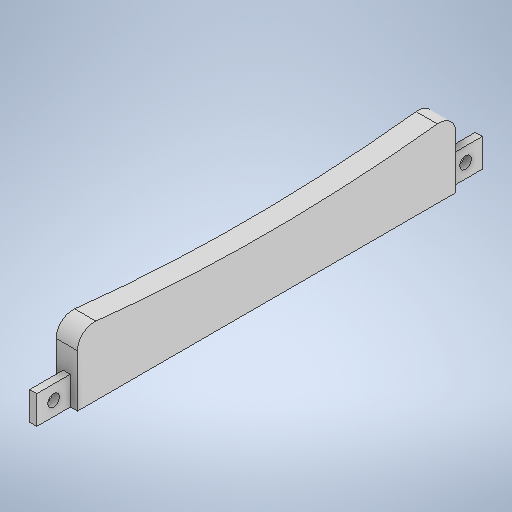
# Autodesk Inventor part: FretBar
Saved by Autodesk Inventor 2025.1 (Build 291241000, 241)
## iProperties
Created: 2025-12-10
Part Number: FretBar
Material: Generic
Document SubType Name: Modeling
Designer: Juxin
Density: 1 g/cm^3
Appearance: Default
Author: Juxin
Title: Fret Bar
Autodesk Inventor part; units mm, degrees
ref_plane "YZ Plane" through (0, 0, 0) normal (1, 0, 0) x (0, 1, 0)
ref_plane "XZ Plane" through (0, 0, 0) normal (0, 1, 0) x (-1, 0, 0)
ref_plane "XY Plane" through (0, 0, 0) normal (0, 0, 1) x (1, 0, 0)
sketch "Sketch1" plane through (0, 0, 0) normal (0, 1, 0) x (-1, 0, 0)
  line L0 (0, 0) -> (1.905, 0)
  line L1 (1.905, -119.6501) -> (0, -119.6501)
  line L2 (0, 0) -> (0, -9.025)
  line L3 (0, 0) -> (9.025, 0) construction
  line L4 (0, -9.025) -> (1.905, -9.025)
  line L5 (0, -119.6501) -> (0, -110.625)
  line L6 (0, -110.625) -> (1.905, -110.625)
  line L7 (1.905, -9.025) -> (3.81, -9.025)
  line L8 (3.81, -9.025) -> (3.81, -110.625)
  line L9 (3.81, -110.625) -> (1.905, -110.625)
  line L10 (0, -9.025) -> (-1.905, -9.025)
  line L11 (-1.905, -9.025) -> (-1.905, -110.625)
  line L12 (-1.905, -110.625) -> (0, -110.625)
  line L13 (1.905, 0) -> (1.905, -9.025)
  line L14 (1.905, -110.625) -> (1.905, -119.6501)
  line L15 (0, -119.6501) -> (0, -110.625)
  line L16 (0, -9.025) -> (0, 0)
  dimension "d19" = 101.6
  dimension "d20" = 1.905
  dimension "d21" = 1.905
  dimension "d22" = 1.905
  dimension "d23" = 1.905
  dimension "d24" = 1.905
  dimension "d25" = 1.905
  constraints: 34 end point, 11 equal length, 9 perpendicular, 4 horizontal, 1 point on line
  measures "d19" distance of L10.end L11.end
  measures "d20" distance of L0.start L0.end
  measures "d21" distance of L4.end L7.end
  measures "d22" distance of L2.end L10.end
  measures "d23" distance of L8.end L6.end
  measures "d24" distance of L11.end L5.end
  measures "d25" distance of L1.start L1.end
extrude "Extrusion1" add sketch "Sketch1" along normal blind 7.62 contours L0 L13 L4 L2 | L6 L14 L1 L5
extrude "Extrusion2" add sketch "Sketch1" along normal blind 19.05 contours L4 L7 L8 L9 L6 L12 L11 L10
sketch "Sketch2" plane through (0, 0, 0) normal (1, 0, 0) x (0, 0, -1)
  line L0 (9.025, 7.62) -> (0, 7.62) projected
  line L1 (4.5125, 7.62) -> (4.5125, 3.81)
  line L2 (0, 0) -> (0, 7.62) projected
  line L3 (9.025, 19.05) -> (110.625, 19.05) projected
  line L4 (59.825, 19.05) -> (59.825, 0)
  line L5 (9.025, 0) -> (110.625, 0) projected
  circle A0 centre (4.5125, 3.81) radius 1.5875
  circle A1 centre (115.1376, 3.81) radius 1.5875
  dimension "d12" = 3.175
  constraints: 4 end point, 3 midpoint, 2 centre point, 1 coincident, 1 parallel, 1 symmetric about line, 1 other
  measures "d12" diameter of A0
extrude "Extrusion3" cut sketch "Sketch2" against normal blind 12.7
sketch "Sketch3" plane through (1.905, 0, -9.025) normal (1, 0, 0) x (0, 0, -1)
  line L0 (0, 19.05) -> (101.6, 19.05) projected
  line L1 (50.8, 19.05) -> (50.8, 15.875)
  arc A0 (0, 19.05) -> (101.6, 19.05) centre (50.8, 423.8625) ccw
  point P0 (-9.025, 0)
  dimension "d15" = 3.175
  constraints: 3 point on circle, 2 end point, 1 centre point, 1 midpoint, 1 vertical
  measures "d15" distance of L1.start L1.end
extrude "Extrusion4" cut sketch "Sketch3" against normal blind 12.7
fillet "Fillet1" radius 4.445 2 edges at (-0.9525, 19.05, -9.025) (-0.9525, 19.05, -110.625)
body "Solid1"
